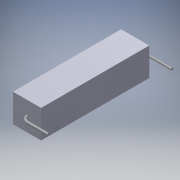
# Autodesk Inventor part: AXIAL-POWER-10W
Saved by Autodesk Inventor 2018.3 (Build 223284000, 284)
## iProperties
Created: 2021-04-19
Part Number: AXIAL-POWER-10W
Material: Genérico
Document SubType Name: Modeling
Designer: laguerre
Density: 8.47 g/cm^3
Appearance: Blanco frío
Author: laguerre
Autodesk Inventor part; units mm, degrees
ref_plane "YZ Plane" through (0, 0, 0) normal (1, 0, 0) x (0, 1, 0)
ref_plane "XZ Plane" through (0, 0, 0) normal (0, 1, 0) x (-1, 0, 0)
ref_plane "XY Plane" through (0, 0, 0) normal (0, 0, 1) x (1, 0, 0)
sketch "Boceto39" plane through (0, 0, 0) normal (0, 0, 1) x (1, 0, 0)
  line L0 (-18.25, 4.75) -> (18.25, 4.75)
  line L1 (18.25, 4.75) -> (18.25, -4.75)
  line L2 (18.25, -4.75) -> (-18.25, -4.75)
  line L3 (-18.25, -4.75) -> (-18.25, 4.75)
  point P0 (0, 0)
  point P1 (0, 4.75)
  point P2 (-18.25, 0)
  dimension "d373" = 36.5
  dimension "d374" = 9.5
  constraints: 8 end point, 2 midpoint, 2 parallel, 1 horizontal, 1 horizontal alignment, 1 perpendicular, 1 vertical alignment
  measures "d373" distance of L0.start L0.end
  measures "d374" distance of L0.end L1.end
extrude "Extrusión13" add sketch "Boceto39" along normal blind 9.5
sketch "Boceto40" plane through (0, 0, 0) normal (0, 1, 0) x (-1, 0, 0)
  line L0 (18.25, 0) -> (-18.25, 0) projected
  line L1 (18.25, 0) -> (18.25, 9.5) projected
  line L2 (-18.25, 9.5) -> (18.25, 9.5) projected
  line L3 (-18.25, 0) -> (-18.25, 9.5) projected
  line L4 (-20, -4.2347) -> (-20, 2.75)
  line L5 (-18, 4.75) -> (18, 4.75)
  line L6 (20, 2.75) -> (20, -6)
  arc A0 (20, 2.75) -> (18, 4.75) centre (18, 2.75) ccw
  arc A1 (-18, 4.75) -> (-20, 2.75) centre (-18, 2.75) ccw
  point P0 (0, 0)
  point P1 (0, 4.75)
  point P2 (18.25, 4.75)
  point P3 (0, 0)
  dimension "d377" = 20
  dimension "d378" = 2
  dimension "d379" = 6
  constraints: 6 end point, 4 point on circle, 4 tangent, 3 midpoint, 2 centre point, 2 perpendicular, 1 equal radius, 1 horizontal alignment, 1 vertical, 1 vertical alignment
  measures "d377" distance from line of point (0, 0) L6
  measures "d378" radius of A0
  measures "d379" distance from line of L0 L6.end
sketch "Boceto41" plane through (0, 0, 0) normal (1, 0, 0) x (0, 1, 0)
  circle A0 centre (0, 4.75) radius 0.4
  point P0 (0, 0)
  dimension "d380" = 0.8
  constraints: 1 centre point, 1 coincident
  measures "d380" diameter of A0
sweep "Barrido1" add profiles "Boceto41" path "Boceto40" path curves L6 A0 L5 A1 L4
